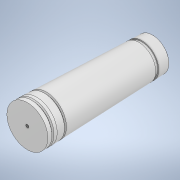
# Autodesk Inventor part: Part1
Saved by Autodesk Inventor 2020.1 (Build 241239000, 239)
## iProperties
Created: 2020-03-27
Part Number: Part1
Material: Aluminum 2014-T6
Document SubType Name: Modeling
Designer: User
Density: 2.78927 g/cm^3
Appearance: Satin
Author: User
Autodesk Inventor part; units mm, degrees
ref_plane "YZ Plane" through (0, 0, 0) normal (1, 0, 0) x (0, 1, 0)
ref_plane "XZ Plane" through (0, 0, 0) normal (0, 1, 0) x (-1, 0, 0)
ref_plane "XY Plane" through (0, 0, 0) normal (0, 0, 1) x (1, 0, 0)
sketch "Sketch1" plane through (0, 0, 0) normal (1, 0, 0) x (0, 1, 0)
  line L0 (-20, 0) -> (122.468, 0)
  line L1 (0, 0) -> (0, -20)
  line L2 (0, -20) -> (9.148, -20)
  line L3 (9.148, -20) -> (122.468, -16.0428)
  line L4 (122.468, 0) -> (122.468, -16.0428)
  line L5 (3, -10) -> (3, -17)
  line L6 (7.8773, 0) -> (3, -10)
  line L7 (7.8773, 0) -> (19.0033, 0) construction
  line L8 (9.2055, 0) -> (9.2055, -16.9852)
  line L9 (8.783, -17) -> (122.468, -13.03)
  line L10 (3, -17) -> (8.783, -17)
  line L11 (122.468, -16.0428) -> (122.3629, -13.0337)
  line L12 (6.0374, -20) -> (4.9651, -19)
  line L13 (4.9651, -19) -> (4.0326, -20)
  line L14 (4.9651, -19) -> (5, -20)
  line L15 (17.532, -19.7072) -> (17.4971, -18.7078)
  line L16 (17.4971, -18.7078) -> (18.5314, -19.6723)
  line L17 (17.4971, -18.7078) -> (16.5326, -19.7421)
  line L18 (111.974, -16.4092) -> (108.9762, -16.5139)
  line L19 (108.9762, -16.5139) -> (108.9413, -15.5145)
  line L20 (108.9413, -15.5145) -> (111.9409, -15.4622)
  line L21 (111.9409, -15.4622) -> (111.974, -16.4092)
  line L22 (0.5, 0) -> (0.5, -1)
  line L23 (0, -1.5) -> (0.5, -1)
  line L24 (0.5, -1) -> (5, -1)
  line L25 (5, -1) -> (5.5774, 0)
  line L26 (0.25, -1.25) -> (4, -1.25)
  line L27 (4, -1.25) -> (4, 0)
  point P0 (4, -1)
  dimension "d1" = 20
  dimension "d5" = 3
  dimension "d18" = 90
  dimension "d22" = 5
  dimension "d23" = 1
  dimension "d24" = 1
  dimension "d25" = 105
  dimension "d26" = 3
  dimension "d27" = 1
  dimension "d28" = 13.5
  dimension "d43" = 88
  constraints: 56 end point, 16 point on line, 6 horizontal, 5 vertical, 4 perpendicular, 1 equal length, 1 midpoint, 1 parallel, 2 other
  measures "d1" distance of L1.start L1.end
  measures "d5" distance between parallel lines of L1 L5
  measures "d18" angle of L13 L12
  measures "d22" distance from line of L1 L14.end
  measures "d23" vertical distance of L12.end L14.end
  measures "d24" distance of L15.start L15.end
  measures "d25" distance between parallel lines of L11 L15
  measures "d26" distance of L19.end L20.end
  measures "d27" distance of L18.end L19.end
  measures "d28" distance between parallel lines of L19 L11
  measures "d43" angle of L3 L4
revolve "Revolution1" add sketch "Sketch1" angle 360 about axis through (0, -20, 0) along (0, 1, 0) contours L23 L26 L27 L24 L25 L0 L6 L5 L10 L9 L11 L3 L21 L20 L19 L16 L17 L2 L12 L13 L1
fillet "Fillet1" radius 0.2 2 edges at (0, 122.468, 16.0428) (0, 122.3629, 13.0337)
thread "Thread2" size "M2.5x0.45" class "6H" standard "ANSI Metric M Profile" length 3.5
move or copy body "Поворот1" bodies to move or copy 1 copy no rotation origin (0, 0, 0) rotation axis (0, 0, 1) rotation angle -90 translate (-65.473, 65.473, 0)
move or copy body "Поворот2" bodies to move or copy 1 copy no rotation origin (0, 0, 0) rotation axis (0, 1, 0) rotation angle 90 translate (56.7951, 0, 56.7951)
body "Solid1"
